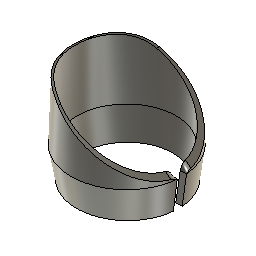
wanner-nose (Autodesk Fusion 360 design; units mm, degrees)
Autodesk Fusion 360 part; units mm, degrees
sketch "Sketch1" plane through (0, 0, 0) normal (0, 0, 1) x (1, 0, 0) in component "wanner-nose"
  arc A0 (14.961, 1.0814) -> (14.9175, -1.5706) centre (0, 0) ccw
  arc A1 (16.9558, 1.2256) -> (16.9181, -1.6665) centre (0, 0) ccw
  line L0 (14.961, 1.0814) -> (16.9558, 1.2256)
  line L1 (16.9181, -1.6665) -> (14.9175, -1.5706)
  dimension "d1" = 15
  dimension "d2" = 17
  constraint coincident A0.centre A1.centre
  measures "d1" radius of A0
  measures "d2" radius of A1
ref_plane "WorkPlane1" through (-0.1274, -0.2024, 10) normal (0, 0, 1) x (1, 0, 0) in component "wanner-nose"
sketch "Sketch3" plane through (-0.1274, -0.2024, 10) normal (0, 0, 1) x (1, 0, 0) in component "wanner-nose"
  arc A0 (16.4407, 1.398) -> (16.4396, -1.4105) centre (0, 0) ccw
  arc A1 (18.4369, 1.5269) -> (18.4325, -1.5793) centre (0, 0) ccw
  line L0 (18.4325, -1.5793) -> (16.4396, -1.4105)
  line L1 (16.4407, 1.398) -> (18.4369, 1.5269)
  dimension "d8" = 16.5
  dimension "d9" = 18.5
  constraint coincident A0.centre A1.centre
  measures "d8" radius of A0
  measures "d9" radius of A1
loft "Loft1" add profiles "Sketch3", "Sketch1" section 1 section 2 in component "wanner-nose"
extrude "Extrude1" add 1 faces at (17.5002, 2.1891, 10) along direction (0, 0, 1) blind 20 draft -2 in component "wanner-nose"
sketch "Sketch4" plane through (0, 0, 0) normal (0, 1, 0) x (1, 0, 0) in component "wanner-nose"
  line L0 (19, -10) -> (-11, -30)
  line L1 (-11, -30) -> (-11, -34)
  line L2 (-11, -34) -> (25.3325, -34)
  line L3 (25.3325, -34) -> (19, -10)
  constraint vertical L1
  constraint perpendicular L1 L2
extrude "Extrude2" cut sketch "Sketch4" along normal blind 35 and the other way blind 46 in component "wanner-nose"
fillet "Fillet1" radius 19.5 2 edges at (-11, -13.913, 30) (-11, 13.5082, 30) in component "wanner-nose"
fillet "Fillet2" radius 2 2 edges at (17.3275, -1.738, 11.115) (17.3304, 1.3003, 11.1131) in component "wanner-nose"
component "wanner-nose" placed x (1, 0, 0) y (0, 1, 0) z (0, 0, 1) at (0, 0, 0)
equation "d1 = ( 30 / 2 ) * 1 mm"
equation "d2 = ( 34 / 2 ) * 1 mm"
equation "d8 = ( 33 / 2 ) * 1 mm"
equation "d9 = ( 37 / 2 ) * 1 mm"
